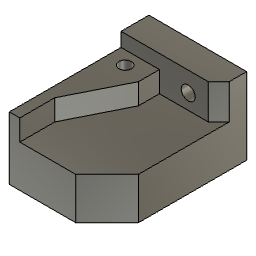
Robocon task1a (Autodesk Fusion 360 design; units mm, degrees)
Autodesk Fusion 360 part; units mm, degrees
note: some values were not read from the file. Set by a fixed rule: which sketch regions a step uses.
sketch "Sketch1" plane through (0, 0, 0) normal (0, 0, 1) x (1, 0, 0)
  line L0 (-75, 100) -> (65, 100)
  line L1 (65, 100) -> (65, -100)
  line L2 (65, -100) -> (-75, -100)
  line L3 (-75, -100) -> (-75, 100)
  line L4 (38.9966, -100) -> (40, -100)
  line L5 (20, -100) -> (65, -55)
  line L6 (-60, -100) -> (-60, -50)
  line L7 (-60, -50) -> (-20, 30)
  line L8 (-20, 30) -> (-20, 60)
  line L9 (-20, 60) -> (50, 60)
  line L10 (50, 60) -> (70, 80)
  line L11 (70, 80) -> (70, 100)
  line L12 (-20, 60) -> (-75, 60)
  constraint horizontal L0
  constraint perpendicular L0 L1
  constraint parallel L0 L2
  constraint parallel L1 L3
  constraint coincident L2 L4.start
  constraint coincident L2 L4.end
  constraint coincident L2 L5.start
  constraint coincident L1 L5.end
  constraint coincident L2 L6.start
  constraint perpendicular L2 L6
  constraint perpendicular L2 L8
  constraint perpendicular L8 L9
  constraint coincident L0 L11.end
  constraint perpendicular L0 L11
  constraint coincident L3 L12.end
  constraint perpendicular L3 L12
extrude "Extrude1" add sketch "Sketch1" along normal blind 20 contours L1 L2 L5 L6 L7 L8 L9 L10
extrude "Extrude2" add sketch "Sketch1" along normal blind 40 contours L2 L3 L6 L7 L8 L12
extrude "Extrude3" add sketch "Sketch1" along normal blind 70 contours L0 L1 L3 L9 L10 L12
sketch "Sketch2" plane through (0, 0, 40) normal (0, 0, 1) x (-1, 0, 0)
  line L0 (60, 100) -> (60, 50)
  line L1 (60, 50) -> (20, -30)
  line L2 (20, -30) -> (20, -60)
  line L3 (20, -60) -> (75, -60)
  line L4 (75, -60) -> (75, 100)
  line L5 (75, 100) -> (60, 100)
  circle A0 centre (50, -41) radius 9.056
sketch "Sketch3" plane through (0, 60, 0) normal (0, -1, 0) x (1, 0, 0)
  line L0 (-75, 40) -> (-20, 40)
  line L1 (-20, 40) -> (-20, 20)
  line L2 (-20, 20) -> (50, 20)
  line L3 (50, 20) -> (50, 70)
  line L4 (50, 70) -> (-75, 70)
  line L5 (-75, 70) -> (-75, 40)
  circle A0 centre (20, 45) radius 11.8346
extrude "Extrude4" add 1 faces at (-5, -25, 20) along direction (0, 0, 1) blind 40
extrude "Extrude5" add sketch "Sketch2" along normal blind 50
extrude "Extrude6" add 1 faces at (-10, 86.6667, 70) along direction (0, 0, 1) blind 40
sketch "Sketch4" plane through (0, 60, 0) normal (0, -1, 0) x (1, 0, 0)
  line L0 (-20, 90) -> (-20, 60)
  line L1 (-20, 60) -> (50, 60)
  line L2 (50, 60) -> (50, 110)
  line L3 (50, 110) -> (-75, 110)
  line L4 (-75, 110) -> (-75, 90)
  line L5 (-75, 90) -> (-20, 90)
hole "Hole1" at (21.3246, 60, 81.6312) direction (0, 1, 0) diameter 20 depth 15 tip angle 180
sketch "Sketch5" plane through (0, 0, 0) normal (0, 0, 1) x (1, 0, 0)
